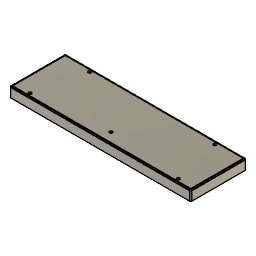
Like Vortex Core (Autodesk Fusion 360 design; units mm, degrees)
Autodesk Fusion 360 part; units mm, degrees
sketch "Sketch1" plane through (0, 0, 0) normal (0, 0, 1) x (1, 0, 0)
  line L0 (40.7197, 73.9331) -> (54.719, 73.9331)
  line L1 (19.0004, 40.8838) -> (5.0009, 40.8838)
  line L2 (173.782, 40.8838) -> (159.782, 40.8838)
  line L3 (238.075, 54.8831) -> (238.075, 40.8838)
  line L4 (54.719, 73.9331) -> (54.719, 59.9338)
  line L5 (245.219, 21.8336) -> (231.22, 21.8336)
  line L6 (40.7197, 59.9338) -> (40.7197, 73.9331)
  line L7 (211.882, 40.8838) -> (197.882, 40.8838)
  line L8 (59.7697, 73.9331) -> (73.769, 73.9331)
  line L9 (83.5822, 54.8831) -> (97.5815, 54.8831)
  line L10 (2.6197, 59.9338) -> (2.6197, 73.9331)
  line L11 (54.719, 59.9338) -> (40.7197, 59.9338)
  line L12 (173.782, 54.8831) -> (173.782, 40.8838)
  line L13 (64.5322, 40.8838) -> (64.5322, 54.8831)
  line L14 (83.5822, 40.8838) -> (83.5822, 54.8831)
  line L15 (21.6697, 59.9338) -> (21.6697, 73.9331)
  line L16 (159.782, 40.8838) -> (159.782, 54.8831)
  line L17 (26.4322, 40.8838) -> (26.4322, 54.8831)
  line L18 (97.5815, 40.8838) -> (83.5822, 40.8838)
  line L19 (245.219, 35.833) -> (245.219, 21.8336)
  line L20 (59.4815, 40.8838) -> (45.4822, 40.8838)
  line L21 (209.787, 35.833) -> (223.788, 35.833)
  line L22 (135.682, 40.8838) -> (121.682, 40.8838)
  line L23 (135.682, 54.8831) -> (135.682, 40.8838)
  line L24 (192.832, 54.8831) -> (192.832, 40.8838)
  line L25 (40.4315, 40.8838) -> (26.4322, 40.8838)
  line L26 (178.832, 40.8838) -> (178.832, 54.8831)
  line L27 (211.882, 54.8831) -> (211.882, 40.8838)
  line L28 (16.6192, 59.9338) -> (2.6196, 59.9338)
  line L29 (231.22, 35.833) -> (245.219, 35.833)
  line L30 (231.22, 21.8336) -> (231.22, 35.833)
  line L31 (16.6192, 73.9331) -> (16.6192, 59.9338)
  line L32 (238.075, 40.8838) -> (224.076, 40.8838)
  line L33 (154.732, 54.8831) -> (154.732, 40.8838)
  line L34 (154.732, 40.8838) -> (140.732, 40.8838)
  line L35 (223.788, 21.8336) -> (209.787, 21.8336)
  line L36 (64.5322, 54.8831) -> (78.5315, 54.8831)
  line L37 (197.882, 54.8831) -> (211.882, 54.8831)
  line L38 (5.0009, 54.8831) -> (19.0004, 54.8831)
  line L39 (21.6697, 73.9331) -> (35.669, 73.9331)
  line L40 (2.6197, 73.9331) -> (16.6192, 73.9331)
  line L41 (140.732, 40.8838) -> (140.732, 54.8831)
  line L42 (35.669, 73.9331) -> (35.669, 59.9338)
  line L43 (192.832, 40.8838) -> (178.832, 40.8838)
  line L44 (188.357, 21.8336) -> (188.357, 35.833)
  line L45 (197.882, 40.8838) -> (197.882, 54.8831)
  line L46 (102.632, 54.8831) -> (116.632, 54.8831)
  line L47 (178.832, 54.8831) -> (192.832, 54.8831)
  line L48 (59.4815, 54.8831) -> (59.4815, 40.8838)
  line L49 (224.076, 54.8831) -> (238.075, 54.8831)
  line L50 (19.0004, 54.8831) -> (19.0004, 40.8838)
  line L51 (133.587, 2.7836) -> (147.588, 2.7836)
  line L52 (45.4822, 40.8838) -> (45.4822, 54.8831)
  line L53 (116.632, 40.8838) -> (102.632, 40.8838)
  line L54 (5.0009, 40.8838) -> (5.0009, 54.8831)
  line L55 (159.782, 54.8831) -> (173.782, 54.8831)
  line L56 (26.4322, 54.8831) -> (40.4315, 54.8831)
  line L57 (97.5815, 54.8831) -> (97.5815, 40.8838)
  line L58 (223.788, 35.833) -> (223.788, 21.8336)
  line L59 (116.632, 54.8831) -> (116.632, 40.8838)
  line L60 (45.4822, 54.8831) -> (59.4815, 54.8831)
  line L61 (78.5315, 40.8838) -> (64.5322, 40.8838)
  line L62 (35.669, 59.9338) -> (21.6697, 59.9338)
  line L63 (209.787, 21.8336) -> (209.787, 35.833)
  line L64 (140.732, 54.8831) -> (154.732, 54.8831)
  line L65 (121.682, 40.8838) -> (121.682, 54.8831)
  line L66 (121.682, 54.8831) -> (135.682, 54.8831)
  line L67 (102.632, 40.8838) -> (102.632, 54.8831)
  line L68 (78.5315, 54.8831) -> (78.5315, 40.8838)
  line L69 (0.0951, 76.4575) -> (247.745, 76.4575)
  line L70 (40.4315, 54.8831) -> (40.4315, 40.8838)
  line L71 (224.076, 40.8838) -> (224.076, 54.8831)
  line L72 (0.0951, 0.2577) -> (0.0951, 76.4575)
  line L73 (247.745, 0.2577) -> (0.0951, 0.2577)
  line L74 (247.745, 76.4575) -> (247.745, 0.2577)
  line L75 (40.4315, 16.7831) -> (40.4315, 2.7836)
  line L76 (59.4815, 2.7836) -> (45.4822, 2.7836)
  line L77 (64.5322, 16.7831) -> (78.5315, 16.7831)
  line L78 (59.4815, 16.7831) -> (59.4815, 2.7836)
  line L79 (45.4822, 2.7836) -> (45.4822, 16.7831)
  line L80 (78.5315, 16.7831) -> (78.5315, 2.7836)
  line L81 (64.5322, 2.7836) -> (64.5322, 16.7831)
  line L82 (35.9572, 21.8336) -> (35.9572, 35.833)
  line L83 (202.357, 2.7836) -> (188.357, 2.7836)
  line L84 (19.0004, 2.7836) -> (5.0009, 2.7836)
  line L85 (90.726, 2.7836) -> (90.726, 16.7831)
  line L86 (5.0009, 16.7831) -> (19.0004, 16.7831)
  line L87 (26.4322, 2.7836) -> (26.4322, 16.7831)
  line L88 (88.0565, 35.833) -> (88.0565, 21.8336)
  line L89 (221.407, 16.7831) -> (221.407, 2.7836)
  line L90 (35.9572, 35.833) -> (49.9565, 35.833)
  line L91 (55.0072, 21.8336) -> (55.0072, 35.833)
  line L92 (147.588, 16.7831) -> (133.587, 16.7831)
  line L93 (45.4822, 16.7831) -> (59.4815, 16.7831)
  line L94 (78.5315, 2.7836) -> (64.5322, 2.7836)
  line L95 (40.4315, 2.7836) -> (26.4322, 2.7836)
  line L96 (19.0004, 16.7831) -> (19.0004, 2.7836)
  line L97 (5.0009, 2.7836) -> (5.0009, 16.7831)
  line L98 (26.4322, 16.7831) -> (40.4315, 16.7831)
  line L99 (9.762, 21.8336) -> (9.762, 35.833)
  line L100 (107.107, 35.833) -> (107.107, 21.8336)
  line L101 (88.0565, 21.8336) -> (74.0572, 21.8336)
  line L102 (49.9565, 21.8336) -> (35.9572, 21.8336)
  line L103 (90.726, 16.7831) -> (104.725, 16.7831)
  line L104 (183.307, 16.7831) -> (183.307, 2.7836)
  line L105 (107.107, 21.8336) -> (93.1072, 21.8336)
  line L106 (188.357, 16.7831) -> (202.357, 16.7831)
  line L107 (112.157, 35.833) -> (126.157, 35.833)
  line L108 (126.157, 21.8336) -> (112.157, 21.8336)
  line L109 (169.307, 2.7836) -> (169.307, 16.7831)
  line L110 (169.307, 16.7831) -> (183.307, 16.7831)
  line L111 (183.307, 2.7836) -> (169.307, 2.7836)
  line L112 (202.357, 16.7831) -> (202.357, 2.7836)
  line L113 (104.725, 2.7836) -> (90.726, 2.7836)
  line L114 (93.1072, 35.833) -> (107.107, 35.833)
  line L115 (131.207, 35.833) -> (145.207, 35.833)
  line L116 (150.257, 21.8336) -> (150.257, 35.833)
  line L117 (164.257, 35.833) -> (164.257, 21.8336)
  line L118 (188.357, 2.7836) -> (188.357, 16.7831)
  line L119 (207.407, 2.7836) -> (207.407, 16.7831)
  line L120 (169.307, 35.833) -> (183.307, 35.833)
  line L121 (69.0065, 21.8336) -> (55.0072, 21.8336)
  line L122 (49.9565, 35.833) -> (49.9565, 21.8336)
  line L123 (126.157, 35.833) -> (126.157, 21.8336)
  line L124 (164.257, 21.8336) -> (150.257, 21.8336)
  line L125 (145.207, 35.833) -> (145.207, 21.8336)
  line L126 (55.0072, 35.833) -> (69.0065, 35.833)
  line L127 (183.307, 35.833) -> (183.307, 21.8336)
  line L128 (112.157, 21.8336) -> (112.157, 35.833)
  line L129 (131.207, 21.8336) -> (131.207, 35.833)
  line L130 (104.725, 16.7831) -> (104.725, 2.7836)
  line L131 (93.1072, 21.8336) -> (93.1072, 35.833)
  line L132 (145.207, 21.8336) -> (131.207, 21.8336)
  line L133 (150.257, 35.833) -> (164.257, 35.833)
  line L134 (242.838, 2.7836) -> (228.837, 2.7836)
  line L135 (221.407, 2.7836) -> (207.407, 2.7836)
  line L136 (69.0065, 35.833) -> (69.0065, 21.8336)
  line L137 (74.0572, 35.833) -> (88.0565, 35.833)
  line L138 (207.407, 16.7831) -> (221.407, 16.7831)
  line L139 (207.119, 59.9338) -> (193.12, 59.9338)
  line L140 (202.357, 35.833) -> (202.357, 21.8336)
  line L141 (23.7629, 21.8336) -> (9.762, 21.8336)
  line L142 (116.918, 73.9331) -> (130.919, 73.9331)
  line L143 (183.307, 21.8336) -> (169.307, 21.8336)
  line L144 (228.837, 16.7831) -> (242.838, 16.7831)
  line L145 (228.837, 2.7836) -> (228.837, 16.7831)
  line L146 (188.357, 35.833) -> (202.357, 35.833)
  line L147 (23.7629, 35.833) -> (23.7629, 21.8336)
  line L148 (242.838, 16.7831) -> (242.838, 2.7836)
  line L149 (74.0572, 21.8336) -> (74.0572, 35.833)
  line L150 (9.762, 35.833) -> (23.7629, 35.833)
  line L151 (202.357, 21.8336) -> (188.357, 21.8336)
  line L152 (169.307, 21.8336) -> (169.307, 35.833)
  line L153 (188.069, 59.9338) -> (174.07, 59.9338)
  line L154 (169.019, 59.9338) -> (155.02, 59.9338)
  line L155 (97.8683, 59.9338) -> (97.8683, 73.9331)
  line L156 (135.97, 73.9331) -> (149.969, 73.9331)
  line L157 (169.019, 73.9331) -> (169.019, 59.9338)
  line L158 (226.169, 73.9331) -> (226.169, 59.9338)
  line L159 (73.769, 59.9338) -> (59.7697, 59.9338)
  line L160 (193.12, 73.9331) -> (207.119, 73.9331)
  line L161 (97.8683, 73.9331) -> (111.869, 73.9331)
  line L162 (155.02, 59.9338) -> (155.02, 73.9331)
  line L163 (111.869, 59.9338) -> (97.8683, 59.9338)
  line L164 (116.918, 59.9338) -> (116.918, 73.9331)
  line L165 (188.069, 73.9331) -> (188.069, 59.9338)
  line L166 (78.8197, 59.9338) -> (78.8197, 73.9331)
  line L167 (155.02, 73.9331) -> (169.019, 73.9331)
  line L168 (73.769, 73.9331) -> (73.769, 59.9338)
  line L169 (149.969, 73.9331) -> (149.969, 59.9338)
  line L170 (174.07, 73.9331) -> (188.069, 73.9331)
  line L171 (59.7697, 59.9338) -> (59.7697, 73.9331)
  line L172 (193.12, 59.9338) -> (193.12, 73.9331)
  line L173 (212.17, 59.9338) -> (212.17, 73.9331)
  line L174 (207.119, 73.9331) -> (207.119, 59.9338)
  line L175 (226.169, 59.9338) -> (212.17, 59.9338)
  line L176 (130.919, 59.9338) -> (116.918, 59.9338)
  line L177 (92.819, 59.9338) -> (78.8197, 59.9338)
  line L178 (130.919, 73.9331) -> (130.919, 59.9338)
  line L179 (149.969, 59.9338) -> (135.97, 59.9338)
  line L180 (78.8197, 73.9331) -> (92.819, 73.9331)
  line L181 (245.219, 59.9338) -> (231.22, 59.9338)
  line L182 (135.97, 59.9338) -> (135.97, 73.9331)
  line L183 (231.22, 73.9331) -> (245.219, 73.9331)
  line L184 (92.819, 73.9331) -> (92.819, 59.9338)
  line L185 (231.22, 59.9338) -> (231.22, 73.9331)
  line L186 (212.17, 73.9331) -> (226.169, 73.9331)
  line L187 (111.869, 73.9331) -> (111.869, 59.9338)
  line L188 (245.219, 73.9331) -> (245.219, 59.9338)
  line L189 (174.07, 59.9338) -> (174.07, 73.9331)
  line L190 (133.587, 16.7831) -> (133.587, 2.7836)
  line L191 (147.588, 2.7836) -> (147.588, 16.7831)
  line L192 (2.1383, 74.6931) -> (2.1383, 1.9601)
  line L193 (2.1383, 1.9601) -> (245.7226, 1.9601)
  line L194 (245.7226, 1.9601) -> (245.7226, 74.6931)
  line L195 (245.7226, 74.6931) -> (2.1383, 74.6931)
  line L196 (221.407, 9.3668) -> (228.837, 9.3668)
  line L197 (228.837, 9.3668) -> (228.837, 1.9601)
  line L198 (228.837, 1.9601) -> (221.407, 1.9601)
  line L199 (221.407, 1.9601) -> (221.407, 9.3668)
  line L200 (19.0004, 9.373) -> (26.4322, 9.373)
  line L201 (26.4322, 9.373) -> (26.4322, 1.9601)
  line L202 (26.4322, 1.9601) -> (19.0004, 1.9601)
  line L203 (19.0004, 1.9601) -> (19.0004, 9.373)
  circle A0 centre (123.9304, 14.9601) radius 3.5951
  line L204 (226.169, 68.4327) -> (231.22, 68.4327)
  line L205 (231.22, 68.4327) -> (231.22, 74.6931)
  line L206 (231.22, 74.6931) -> (226.169, 74.6931)
  line L207 (226.169, 74.6931) -> (226.169, 68.4327)
  line L208 (16.6192, 68.371) -> (21.6697, 68.371)
  line L209 (21.6697, 68.371) -> (21.6697, 74.6931)
  line L210 (21.6697, 74.6931) -> (16.6192, 74.6931)
  line L211 (16.6192, 74.6931) -> (16.6192, 68.371)
  line L212 (212.17, 68.3537) -> (207.119, 68.3537)
  line L213 (207.119, 73.9331) -> (207.119, 74.6931)
  line L214 (212.17, 73.9331) -> (212.17, 74.6931)
  line L215 (35.669, 68.3674) -> (40.7197, 68.3674)
  line L216 (40.7197, 73.9331) -> (40.7197, 74.6931)
  line L217 (35.669, 73.9331) -> (35.669, 74.6931)
  constraint perpendicular L51 L190
  constraint perpendicular L92 L191
  constraint perpendicular L73 L192
  constraint perpendicular L74 L193
  constraint perpendicular L193 L194
  constraint perpendicular L192 L195
  constraint parallel L69 L195
  constraint parallel L72 L192
  constraint parallel L73 L193
  constraint horizontal L196
  constraint vertical L197
  constraint horizontal L198
  constraint vertical L199
  constraint coincident L193 L197.end
  constraint coincident L89 L196.start
  constraint horizontal L200
  constraint vertical L201
  constraint horizontal L202
  constraint vertical L203
  constraint coincident L193 L201.end
  constraint coincident L96 L200.start
  constraint horizontal L204
  constraint vertical L205
  constraint horizontal L206
  constraint vertical L207
  constraint coincident L195 L205.end
  constraint coincident L158 L204.start
  constraint horizontal L208
  constraint vertical L209
  constraint horizontal L210
  constraint vertical L211
  constraint coincident L195 L209.end
  constraint coincident L31 L208.start
  constraint coincident L173 L212.start
  constraint coincident L174 L212.end
  constraint perpendicular L174 L212
  constraint coincident L195 L213.end
  constraint perpendicular L195 L213
  constraint coincident L195 L214.end
  constraint perpendicular L195 L214
  constraint coincident L42 L215.start
  constraint coincident L6 L215.end
  constraint perpendicular L6 L215
  constraint coincident L195 L216.end
  constraint perpendicular L195 L216
  constraint coincident L195 L217.end
  constraint perpendicular L195 L217
extrude "Extrude1" add sketch "Sketch1" against normal blind 1.5 contours L0 L4 L6 L10 L11 L15 L28 L31 L40 L42 L62 L75 L84 L86 L87 L89 L95 L96 L97 L98 L119 L134 L135 L138 L139 L144 L145 L148 L158 L160 L172 L173 L174 L175 L181 L183 L185 L188 L192 L193 L194 L195 L196 L197 L199 L200 L201 L203 L204 L205 L208 L211 L212 L213 L215 L216 | L6 L42 L195 L215 L216 L217 | L173 L174 L195 L212 L213 L214 | L39 L195 L209 L217 | L186 L195 L207 L214 | L15 L31 L195 L208 L209 L210 L211 | L158 L185 L195 L204 L205 L206 L207 | L87 L96 L193 L200 L201 L202 L203 | L89 L145 L193 L196 L197 L198 L199 | L69 L72 L73 L74 | A0 makes body 1
extrude "Extrude2" add sketch "Sketch1" along normal blind 3.5 contours L69 L72 L73 L74 bodies 1
extrude "Extrude6" add 1 faces at (0.7761, 50.4694, 3.5) along direction (0, 0, 1) blind 7.5 draft 10 on bodies 1 bodies 1
sketch "Sketch6" plane through (0, 0, -1.5) normal (0, 0, -1) x (1, 0, 0)
  line L0 (147.588, -2.7836) -> (147.588, -16.7831)
  line L1 (147.588, -16.7831) -> (133.587, -16.7831)
  line L2 (133.587, -16.7831) -> (133.587, -2.7836)
  line L3 (133.587, -2.7836) -> (147.588, -2.7836)
  line L4 (174.07, -59.9338) -> (188.069, -59.9338)
  line L5 (188.069, -59.9338) -> (188.069, -73.9331)
  line L6 (188.069, -73.9331) -> (174.07, -73.9331)
  line L7 (174.07, -73.9331) -> (174.07, -59.9338)
  line L8 (245.219, -73.9331) -> (231.22, -73.9331)
  line L9 (231.22, -73.9331) -> (231.22, -59.9338)
  line L10 (231.22, -59.9338) -> (245.219, -59.9338)
  line L11 (245.219, -59.9338) -> (245.219, -73.9331)
  line L12 (111.869, -73.9331) -> (97.8683, -73.9331)
  line L13 (97.8683, -73.9331) -> (97.8683, -59.9338)
  line L14 (97.8683, -59.9338) -> (111.869, -59.9338)
  line L15 (111.869, -59.9338) -> (111.869, -73.9331)
  line L16 (212.17, -73.9331) -> (212.17, -59.9338)
  line L17 (212.17, -59.9338) -> (226.169, -59.9338)
  line L18 (226.169, -59.9338) -> (226.169, -73.9331)
  line L19 (226.169, -73.9331) -> (212.17, -73.9331)
  line L20 (92.819, -73.9331) -> (78.8197, -73.9331)
  line L21 (78.8197, -73.9331) -> (78.8197, -59.9338)
  line L22 (78.8197, -59.9338) -> (92.819, -59.9338)
  line L23 (92.819, -59.9338) -> (92.819, -73.9331)
  line L24 (135.97, -59.9338) -> (149.969, -59.9338)
  line L25 (149.969, -59.9338) -> (149.969, -73.9331)
  line L26 (149.969, -73.9331) -> (135.97, -73.9331)
  line L27 (135.97, -73.9331) -> (135.97, -59.9338)
  line L28 (130.919, -73.9331) -> (116.918, -73.9331)
  line L29 (116.918, -73.9331) -> (116.918, -59.9338)
  line L30 (116.918, -59.9338) -> (130.919, -59.9338)
  line L31 (130.919, -59.9338) -> (130.919, -73.9331)
  line L32 (207.119, -73.9331) -> (193.12, -73.9331)
  line L33 (193.12, -73.9331) -> (193.12, -59.9338)
  line L34 (193.12, -59.9338) -> (207.119, -59.9338)
  line L35 (207.119, -59.9338) -> (207.119, -73.9331)
  line L36 (59.7697, -59.9338) -> (73.769, -59.9338)
  line L37 (73.769, -59.9338) -> (73.769, -73.9331)
  line L38 (73.769, -73.9331) -> (59.7697, -73.9331)
  line L39 (59.7697, -73.9331) -> (59.7697, -59.9338)
  line L40 (155.02, -73.9331) -> (155.02, -59.9338)
  line L41 (155.02, -59.9338) -> (169.019, -59.9338)
  line L42 (169.019, -59.9338) -> (169.019, -73.9331)
  line L43 (169.019, -73.9331) -> (155.02, -73.9331)
  line L44 (169.307, -21.8336) -> (183.307, -21.8336)
  line L45 (183.307, -21.8336) -> (183.307, -35.833)
  line L46 (183.307, -35.833) -> (169.307, -35.833)
  line L47 (169.307, -35.833) -> (169.307, -21.8336)
  line L48 (202.357, -21.8336) -> (202.357, -35.833)
  line L49 (202.357, -35.833) -> (188.357, -35.833)
  line L50 (188.357, -35.833) -> (188.357, -21.8336)
  line L51 (188.357, -21.8336) -> (202.357, -21.8336)
  line L52 (9.762, -35.833) -> (9.762, -21.8336)
  line L53 (9.762, -21.8336) -> (23.7629, -21.8336)
  line L54 (23.7629, -21.8336) -> (23.7629, -35.833)
  line L55 (23.7629, -35.833) -> (9.762, -35.833)
  line L56 (74.0572, -21.8336) -> (88.0565, -21.8336)
  line L57 (88.0565, -21.8336) -> (88.0565, -35.833)
  line L58 (88.0565, -35.833) -> (74.0572, -35.833)
  line L59 (74.0572, -35.833) -> (74.0572, -21.8336)
  line L60 (242.838, -16.7831) -> (228.837, -16.7831)
  line L61 (228.837, -16.7831) -> (228.837, -2.7836)
  line L62 (228.837, -2.7836) -> (242.838, -2.7836)
  line L63 (242.838, -2.7836) -> (242.838, -16.7831)
  line L64 (207.407, -16.7831) -> (207.407, -2.7836)
  line L65 (207.407, -2.7836) -> (221.407, -2.7836)
  line L66 (221.407, -2.7836) -> (221.407, -16.7831)
  line L67 (221.407, -16.7831) -> (207.407, -16.7831)
  line L68 (69.0065, -35.833) -> (55.0072, -35.833)
  line L69 (55.0072, -35.833) -> (55.0072, -21.8336)
  line L70 (55.0072, -21.8336) -> (69.0065, -21.8336)
  line L71 (69.0065, -21.8336) -> (69.0065, -35.833)
  line L72 (121.682, -54.8831) -> (121.682, -40.8838)
  line L73 (121.682, -40.8838) -> (135.682, -40.8838)
  line L74 (135.682, -40.8838) -> (135.682, -54.8831)
  line L75 (135.682, -54.8831) -> (121.682, -54.8831)
  line L76 (45.4822, -16.7831) -> (45.4822, -2.7836)
  line L77 (45.4822, -2.7836) -> (59.4815, -2.7836)
  line L78 (59.4815, -2.7836) -> (59.4815, -16.7831)
  line L79 (59.4815, -16.7831) -> (45.4822, -16.7831)
  line L80 (183.307, -2.7836) -> (183.307, -16.7831)
  line L81 (183.307, -16.7831) -> (169.307, -16.7831)
  line L82 (169.307, -16.7831) -> (169.307, -2.7836)
  line L83 (169.307, -2.7836) -> (183.307, -2.7836)
  line L84 (93.1072, -21.8336) -> (107.107, -21.8336)
  line L85 (107.107, -21.8336) -> (107.107, -35.833)
  line L86 (107.107, -35.833) -> (93.1072, -35.833)
  line L87 (93.1072, -35.833) -> (93.1072, -21.8336)
  line L88 (45.4822, -54.8831) -> (45.4822, -40.8838)
  line L89 (45.4822, -40.8838) -> (59.4815, -40.8838)
  line L90 (59.4815, -40.8838) -> (59.4815, -54.8831)
  line L91 (59.4815, -54.8831) -> (45.4822, -54.8831)
  line L92 (40.4315, -54.8831) -> (26.4322, -54.8831)
  line L93 (26.4322, -54.8831) -> (26.4322, -40.8838)
  line L94 (26.4322, -40.8838) -> (40.4315, -40.8838)
  line L95 (40.4315, -40.8838) -> (40.4315, -54.8831)
  line L96 (231.22, -21.8336) -> (245.219, -21.8336)
  line L97 (245.219, -21.8336) -> (245.219, -35.833)
  line L98 (245.219, -35.833) -> (231.22, -35.833)
  line L99 (231.22, -35.833) -> (231.22, -21.8336)
  line L100 (104.725, -16.7831) -> (90.726, -16.7831)
  line L101 (90.726, -16.7831) -> (90.726, -2.7836)
  line L102 (90.726, -2.7836) -> (104.725, -2.7836)
  line L103 (104.725, -2.7836) -> (104.725, -16.7831)
  line L104 (150.257, -35.833) -> (150.257, -21.8336)
  line L105 (150.257, -21.8336) -> (164.257, -21.8336)
  line L106 (164.257, -21.8336) -> (164.257, -35.833)
  line L107 (164.257, -35.833) -> (150.257, -35.833)
  line L108 (54.719, -59.9338) -> (54.719, -73.9331)
  line L109 (54.719, -73.9331) -> (40.7197, -73.9331)
  line L110 (40.7197, -73.9331) -> (40.7197, -59.9338)
  line L111 (40.7197, -59.9338) -> (54.719, -59.9338)
  line L112 (35.669, -59.9338) -> (35.669, -73.9331)
  line L113 (35.669, -73.9331) -> (21.6697, -73.9331)
  line L114 (21.6697, -73.9331) -> (21.6697, -59.9338)
  line L115 (21.6697, -59.9338) -> (35.669, -59.9338)
  line L116 (2.6197, -73.9331) -> (2.6197, -59.9338)
  line L117 (2.6197, -59.9338) -> (16.6192, -59.9338)
  line L118 (16.6192, -59.9338) -> (16.6192, -73.9331)
  line L119 (16.6192, -73.9331) -> (2.6197, -73.9331)
  line L120 (159.782, -54.8831) -> (159.782, -40.8838)
  line L121 (159.782, -40.8838) -> (173.782, -40.8838)
  line L122 (173.782, -40.8838) -> (173.782, -54.8831)
  line L123 (173.782, -54.8831) -> (159.782, -54.8831)
  line L124 (145.207, -21.8336) -> (145.207, -35.833)
  line L125 (145.207, -35.833) -> (131.207, -35.833)
  line L126 (131.207, -35.833) -> (131.207, -21.8336)
  line L127 (131.207, -21.8336) -> (145.207, -21.8336)
  line L128 (49.9565, -35.833) -> (35.9572, -35.833)
  line L129 (35.9572, -35.833) -> (35.9572, -21.8336)
  line L130 (35.9572, -21.8336) -> (49.9565, -21.8336)
  line L131 (49.9565, -21.8336) -> (49.9565, -35.833)
  line L132 (178.832, -54.8831) -> (178.832, -40.8838)
  line L133 (178.832, -40.8838) -> (192.832, -40.8838)
  line L134 (192.832, -40.8838) -> (192.832, -54.8831)
  line L135 (192.832, -54.8831) -> (178.832, -54.8831)
  line L136 (5.0009, -40.8838) -> (19.0004, -40.8838)
  line L137 (19.0004, -40.8838) -> (19.0004, -54.8831)
  line L138 (19.0004, -54.8831) -> (5.0009, -54.8831)
  line L139 (5.0009, -54.8831) -> (5.0009, -40.8838)
  line L140 (224.076, -40.8838) -> (238.075, -40.8838)
  line L141 (238.075, -40.8838) -> (238.075, -54.8831)
  line L142 (238.075, -54.8831) -> (224.076, -54.8831)
  line L143 (224.076, -54.8831) -> (224.076, -40.8838)
  line L144 (112.157, -21.8336) -> (126.157, -21.8336)
  line L145 (126.157, -21.8336) -> (126.157, -35.833)
  line L146 (126.157, -35.833) -> (112.157, -35.833)
  line L147 (112.157, -35.833) -> (112.157, -21.8336)
  line L148 (5.0009, -2.7836) -> (19.0004, -2.7836)
  line L149 (19.0004, -2.7836) -> (19.0004, -16.7831)
  line L150 (19.0004, -16.7831) -> (5.0009, -16.7831)
  line L151 (5.0009, -16.7831) -> (5.0009, -2.7836)
  line L152 (78.5315, -2.7836) -> (78.5315, -16.7831)
  line L153 (78.5315, -16.7831) -> (64.5322, -16.7831)
  line L154 (64.5322, -16.7831) -> (64.5322, -2.7836)
  line L155 (64.5322, -2.7836) -> (78.5315, -2.7836)
  line L156 (102.632, -40.8838) -> (116.632, -40.8838)
  line L157 (116.632, -40.8838) -> (116.632, -54.8831)
  line L158 (116.632, -54.8831) -> (102.632, -54.8831)
  line L159 (102.632, -54.8831) -> (102.632, -40.8838)
  line L160 (197.882, -40.8838) -> (211.882, -40.8838)
  line L161 (211.882, -40.8838) -> (211.882, -54.8831)
  line L162 (211.882, -54.8831) -> (197.882, -54.8831)
  line L163 (197.882, -54.8831) -> (197.882, -40.8838)
  line L164 (97.5815, -54.8831) -> (83.5822, -54.8831)
  line L165 (83.5822, -54.8831) -> (83.5822, -40.8838)
  line L166 (83.5822, -40.8838) -> (97.5815, -40.8838)
  line L167 (97.5815, -40.8838) -> (97.5815, -54.8831)
  line L168 (26.4322, -16.7831) -> (26.4322, -2.7836)
  line L169 (26.4322, -2.7836) -> (40.4315, -2.7836)
  line L170 (40.4315, -2.7836) -> (40.4315, -16.7831)
  line L171 (40.4315, -16.7831) -> (26.4322, -16.7831)
  line L172 (188.357, -2.7836) -> (202.357, -2.7836)
  line L173 (202.357, -2.7836) -> (202.357, -16.7831)
  line L174 (202.357, -16.7831) -> (188.357, -16.7831)
  line L175 (188.357, -16.7831) -> (188.357, -2.7836)
  line L176 (209.787, -21.8336) -> (223.788, -21.8336)
  line L177 (223.788, -21.8336) -> (223.788, -35.833)
  line L178 (223.788, -35.833) -> (209.787, -35.833)
  line L179 (209.787, -35.833) -> (209.787, -21.8336)
  line L180 (78.5315, -54.8831) -> (64.5322, -54.8831)
  line L181 (64.5322, -54.8831) -> (64.5322, -40.8838)
  line L182 (64.5322, -40.8838) -> (78.5315, -40.8838)
  line L183 (78.5315, -40.8838) -> (78.5315, -54.8831)
  line L184 (140.732, -54.8831) -> (140.732, -40.8838)
  line L185 (140.732, -40.8838) -> (154.732, -40.8838)
  line L186 (154.732, -40.8838) -> (154.732, -54.8831)
  line L187 (154.732, -54.8831) -> (140.732, -54.8831)
  line L188 (0.0951, -76.4575) -> (247.745, -76.4575)
  line L189 (247.745, -76.4575) -> (247.745, -0.2577)
  line L190 (247.745, -0.2577) -> (0.0951, -0.2577)
  line L191 (0.0951, -0.2577) -> (0.0951, -76.4575)
  line L192 (0.0951, -76.4575) -> (247.745, -76.4575)
  line L193 (247.745, -76.4575) -> (247.745, -0.2577)
  line L194 (247.745, -0.2577) -> (0.0951, -0.2577)
  line L195 (0.0951, -0.2577) -> (0.0951, -76.4575)
  constraint horizontal L192
  constraint vertical L193
  constraint horizontal L194
  constraint vertical L195
  constraint coincident L189.end L190.start
  constraint coincident L188.start L191.end
extrude "Extrude7" cut sketch "Sketch6" against normal blind 40 contours L0 L1 L2 L3 | L4 L5 L6 L7 | L8 L9 L10 L11 | L12 L13 L14 L15 | L16 L17 L18 L19 | L20 L21 L22 L23 | L24 L25 L26 L27 | L28 L29 L30 L31 | L32 L33 L34 L35 | L36 L37 L38 L39 | L40 L41 L42 L43 | L44 L45 L46 L47 | L48 L49 L50 L51 | L52 L53 L54 L55 | L56 L57 L58 L59 | L60 L61 L62 L63 | L64 L65 L66 L67 | L68 L69 L70 L71 | L72 L73 L74 L75 | L76 L77 L78 L79 | L80 L81 L82 L83 | L84 L85 L86 L87 | L88 L89 L90 L91 | L92 L93 L94 L95 | L96 L97 L98 L99 | L100 L101 L102 L103 | L104 L105 L106 L107 | L108 L109 L110 L111 | L112 L113 L114 L115 | L116 L117 L118 L119 | L120 L121 L122 L123 | L124 L125 L126 L127 | L128 L129 L130 L131 | L132 L133 L134 L135 | L136 L137 L138 L139 | L140 L141 L142 L143 | L144 L145 L146 L147 | L148 L149 L150 L151 | L152 L153 L154 L155 | L156 L157 L158 L159 | L160 L161 L162 L163 | L164 L165 L166 L167 | L168 L169 L170 L171 | L172 L173 L174 L175 | L176 L177 L178 L179 | L180 L181 L182 L183 | L184 L185 L186 L187 | L188 L189 L190 L191 L192 L193 L194 L195 keep common part bodies 1
extrude "Extrude4" add sketch "Sketch1" along normal blind 11 contours L6 L42 L195 L215 L216 L217 | L173 L174 L195 L212 L213 L214 | L87 L96 L193 L200 L201 L202 L203 | L89 L145 L193 L196 L197 L198 L199 | A0 bodies 1
sketch "Sketch5" plane through (0, 0, 11) normal (0, 0, 1) x (-1, 0, 0)
  line L0 (-228.837, -3.2826) -> (-228.837, -9.3668)
  line L1 (-228.837, -9.3668) -> (-221.407, -9.3668)
  line L2 (-221.407, -9.3668) -> (-221.407, -3.2826)
  line L3 (-26.4322, -3.2826) -> (-26.4322, -9.373)
  line L4 (-26.4322, -9.373) -> (-19.0004, -9.373)
  line L5 (-19.0004, -9.373) -> (-19.0004, -3.2826)
  line L6 (-247.745, -76.4575) -> (-0.0951, -76.4575)
  line L7 (-0.0951, -76.4575) -> (-0.0951, -0.2577)
  line L8 (-0.0951, -0.2577) -> (-247.745, -0.2577)
  line L9 (-247.745, -0.2577) -> (-247.745, -76.4575)
  line L10 (-2.1277, -74.4552) -> (-245.6919, -74.4552)
  line L11 (-245.6919, -74.4552) -> (-245.6919, -2.3183)
  line L12 (-245.6919, -2.3183) -> (-2.1277, -2.3183)
  line L13 (-2.1277, -2.3183) -> (-2.1277, -74.4552)
  line L14 (-19.0004, -3.2826) -> (-3.4607, -3.2826)
  line L15 (-3.4607, -3.2826) -> (-3.4607, -73.3706)
  line L16 (-40.7197, -73.3706) -> (-207.119, -73.3706)
  line L17 (-244.4001, -73.3706) -> (-244.4001, -3.2826)
  line L18 (-244.4001, -3.2826) -> (-228.837, -3.2826)
  line L19 (-221.407, -3.2826) -> (-26.4322, -3.2826)
  line L20 (-207.119, -73.3706) -> (-207.119, -68.3537)
  line L21 (-207.119, -68.3537) -> (-212.17, -68.3537)
  line L22 (-212.17, -68.3537) -> (-212.17, -73.3706)
  line L23 (-212.17, -73.3706) -> (-244.4001, -73.3706)
  line L24 (-3.4607, -73.3706) -> (-35.669, -73.3706)
  line L25 (-35.669, -73.3706) -> (-35.669, -68.3674)
  line L26 (-35.669, -68.3674) -> (-40.7197, -68.3674)
  line L27 (-40.7197, -68.3674) -> (-40.7197, -73.3706)
  constraint horizontal L10
  constraint vertical L11
  constraint horizontal L12
  constraint vertical L13
extrude "Extrude5" add sketch "Sketch5" along normal blind 1.5 contours L6 L7 L8 L9 bodies 1
fillet "Fillet3" radius 1.5 4 edges at (0.0951, 76.4575, 5.5) (0.0951, 0.2577, 5.5) (247.745, 0.2577, 5.5) (247.745, 76.4575, 5.5) on bodies 1
fillet "Fillet4" radius 19.75 12 edges at (123.9196, 1.9601, 3.5) (237.2798, 1.9601, 3.5) (245.7226, 38.3266, 3.5) (228.9463, 74.6931, 3.5) (123.9194, 74.6931, 3.5) (18.9036, 74.6931, 3.5) (228.9463, 74.6931, 3.5) (123.9194, 74.6931, 3.5) (18.9036, 74.6931, 3.5) (2.1383, 38.3266, 3.5) (18.9036, 74.6931, 3.5) (10.5693, 1.9601, 3.5) on bodies 1
sketch "Sketch7" plane through (0, 76.4575, 0) normal (0, 1, 0) x (-1, 0, 0)
  line L0 (-246.245, 12.5) -> (-246.245, -1.5)
  line L1 (-246.245, -1.5) -> (-1.5951, -1.5)
  line L2 (-1.5951, -1.5) -> (-1.5951, 12.5)
  line L3 (-1.5951, 12.5) -> (-246.245, 12.5)
  line L4 (-23.4098, 9) -> (-14.4098, 9)
  line L5 (-14.4098, 9) -> (-14.4098, 5.5)
  line L6 (-14.4098, 5.5) -> (-23.4098, 5.5)
  line L7 (-23.4098, 5.5) -> (-23.4098, 9)
  line L8 (-245.6919, 11) -> (-2.1277, 11)
  dimension "d27" = 3.5
  constraint horizontal L4
  constraint vertical L5
  constraint horizontal L6
  constraint vertical L7
  measures "d27" distance of L4.start L6.end
extrude "Extrude8" cut sketch "Sketch7" against normal blind 12 contours L4 L5 L6 L7 bodies 1
fillet "Fillet5" radius 1.75 4 edges at (14.4098, 75.0904, 9) (14.4098, 75.3989, 5.5) (23.4098, 75.3989, 5.5) (23.4098, 75.0904, 9) on bodies 1
sketch "Sketch8" plane through (0, 0, 12.5) normal (0, 0, 1) x (-1, 0, 0)
  line L0 (-245.6919, -2.3183) -> (-2.1277, -2.3183)
  line L1 (-2.1277, -2.3183) -> (-2.1277, -74.4552)
  line L2 (-2.1277, -74.4552) -> (-245.6919, -74.4552)
  line L3 (-245.6919, -74.4552) -> (-245.6919, -2.3183)
  arc A0 (-247.745, -74.9575) -> (-246.245, -76.4575) centre (-246.245, -74.9575) ccw
  line L4 (-246.245, -76.4575) -> (-1.5951, -76.4575)
  arc A1 (-1.5951, -76.4575) -> (-0.0951, -74.9575) centre (-1.5951, -74.9575) ccw
  line L5 (-0.0951, -74.9575) -> (-0.0951, -1.7577)
  arc A2 (-0.0951, -1.7577) -> (-1.5951, -0.2577) centre (-1.5951, -1.7577) ccw
  line L6 (-1.5951, -0.2577) -> (-246.245, -0.2577)
  arc A3 (-246.245, -0.2577) -> (-247.745, -1.7577) centre (-246.245, -1.7577) ccw
  line L7 (-247.745, -1.7577) -> (-247.745, -74.9575)
  line L8 (-30.4503, -74.4552) -> (-7.3693, -74.4552)
  line L9 (-7.3693, -74.4552) -> (-7.3693, -67.7003)
  line L10 (-7.3693, -67.7003) -> (-30.4503, -67.7003)
  line L11 (-30.4503, -67.7003) -> (-30.4503, -74.4552)
extrude "Extrude9" cut sketch "Sketch8" against normal blind 12 contours L2 L8 L9 L10 L11 bodies 1
fillet "Fillet6" radius 0.75 4 edges at (2.1277, 74.4552, 11.75) (245.6919, 74.4552, 11.75) (245.6919, 2.3183, 11.75) (2.1277, 2.3183, 11.75) on bodies 1
fillet "Fillet7" radius 1 12 edges at (2.1383, 74.6931, 0.886) (2.2134, 74.6179, 3.4934) (2.9495, 73.8818, 8.1008) (2.1383, 1.9601, 0.886) (2.2134, 2.0353, 3.4934) (2.9495, 2.7714, 8.1008) (245.7226, 1.9601, 0.886) (245.6474, 2.0353, 3.4934) (244.9114, 2.7714, 8.1008) (245.7226, 74.6931, 0.886) (245.6474, 74.6179, 3.4934) (244.9114, 73.8818, 8.1008) on bodies 1
sketch "Sketch11" plane through (0, 0, 12.5) normal (0, 0, 1) x (-1, 0, 0)
  line L0 (-244.9419, -2.3183) -> (-2.8777, -2.3183)
  arc A0 (-2.1277, -3.0683) -> (-2.8777, -2.3183) centre (-2.8777, -3.0683) ccw
  line L1 (-2.1277, -3.0683) -> (-2.1277, -73.7052)
  arc A1 (-2.8777, -74.4552) -> (-2.1277, -73.7052) centre (-2.8777, -73.7052) ccw
  line L2 (-2.8777, -74.4552) -> (-244.9419, -74.4552)
  arc A2 (-245.6919, -73.7052) -> (-244.9419, -74.4552) centre (-244.9419, -73.7052) ccw
  line L3 (-245.6919, -73.7052) -> (-245.6919, -3.0683)
  arc A3 (-244.9419, -2.3183) -> (-245.6919, -3.0683) centre (-244.9419, -3.0683) ccw
  arc A4 (-247.745, -74.9575) -> (-246.245, -76.4575) centre (-246.245, -74.9575) ccw
  line L4 (-246.245, -76.4575) -> (-1.5951, -76.4575)
  arc A5 (-1.5951, -76.4575) -> (-0.0951, -74.9575) centre (-1.5951, -74.9575) ccw
  line L5 (-0.0951, -74.9575) -> (-0.0951, -1.7577)
  arc A6 (-0.0951, -1.7577) -> (-1.5951, -0.2577) centre (-1.5951, -1.7577) ccw
  line L6 (-1.5951, -0.2577) -> (-246.245, -0.2577)
  arc A7 (-246.245, -0.2577) -> (-247.745, -1.7577) centre (-246.245, -1.7577) ccw
  line L7 (-247.745, -1.7577) -> (-247.745, -74.9575)
extrude "Extrude10" add sketch "Sketch11" against normal blind 1.5 separate body contours L0 A0 L1 A1 L2 A2 L3 A3 makes body 2
sketch "Sketch12" plane through (0, 0, 11) normal (0, 0, -1) x (1, 0, 0)
  arc A0 (2.8777, -2.3183) -> (2.1277, -3.0683) centre (2.8777, -3.0683) ccw
  line L0 (2.1277, -3.0683) -> (2.1277, -73.7052)
  arc A1 (2.1277, -73.7052) -> (2.8777, -74.4552) centre (2.8777, -73.7052) ccw
  line L1 (2.8777, -74.4552) -> (244.9419, -74.4552)
  arc A2 (244.9419, -74.4552) -> (245.6919, -73.7052) centre (244.9419, -73.7052) ccw
  line L2 (245.6919, -73.7052) -> (245.6919, -3.0683)
  arc A3 (245.6919, -3.0683) -> (244.9419, -2.3183) centre (244.9419, -3.0683) ccw
  line L3 (244.9419, -2.3183) -> (2.8777, -2.3183)
  line L4 (30.4098, -74.4552) -> (7.4098, -74.4552)
  line L5 (7.4098, -74.4552) -> (7.4098, -37.4552)
  line L6 (7.4098, -37.4552) -> (30.4098, -37.4552)
  line L7 (30.4098, -37.4552) -> (30.4098, -74.4552)
  line L8 (32.3439, -74.4552) -> (5.4296, -74.4552)
  line L9 (5.4296, -74.4552) -> (5.4296, -35.2609)
  line L10 (5.4296, -35.2609) -> (32.3439, -35.2609)
  line L11 (32.3439, -35.2609) -> (32.3439, -74.4552)
  line L12 (7.4098, -37.4552) -> (7.4098, -35.2609)
  line L13 (30.4098, -37.4552) -> (30.4098, -35.2609)
  dimension "d44" = 23
  dimension "d45" = 37
  constraint horizontal L4
  constraint vertical L5
  constraint horizontal L6
  constraint vertical L7
  constraint coincident L1 L4.start
  constraint horizontal L8
  constraint vertical L9
  constraint horizontal L10
  constraint vertical L11
  constraint coincident L1 L8.start
  constraint coincident L10 L12.end
  constraint perpendicular L10 L12
  constraint coincident L10 L13.end
  constraint perpendicular L10 L13
  measures "d44" distance of L4.start L4.end
  measures "d45" distance of L4.start L6.end
extrude "Extrude11" add sketch "Sketch12" along normal blind 2 contours L6 L10 L12 L13 bodies 2
fillet "Fillet10" radius 1 8 edges at (247.3057, 76.0182, 12.5) (123.92, 76.4575, 12.5) (0.5344, 76.0182, 12.5) (0.0951, 38.3576, 12.5) (0.5344, 0.697, 12.5) (123.92, 0.2577, 12.5) (247.3057, 0.697, 12.5) (247.745, 38.3576, 12.5) on bodies 1
fillet "Fillet11" radius 1 5 edges at (120.5786, 16.2602, 0) (225.122, 9.3668, 0) (22.7163, 9.373, 0) (209.6445, 68.3537, 0) (38.1944, 68.3674, 0) on bodies 1
fillet "Fillet12" radius 0.75 24 edges at (212.17, 73.8818, 8.1008) (212.17, 74.6179, 3.4934) (212.17, 74.6931, 0.886) (207.119, 74.6931, 0.886) (207.119, 74.6179, 3.4934) (207.119, 73.8818, 8.1008) (40.7197, 73.8818, 8.1008) (40.7197, 74.6179, 3.4934) (40.7197, 74.6931, 0.886) (35.669, 74.6931, 0.886) (35.669, 74.6179, 3.4934) (35.669, 73.8818, 8.1008) (26.4322, 1.9601, 0.886) (26.4322, 2.0353, 3.4934) (26.4322, 2.7714, 8.1008) (19.0004, 2.7714, 8.1008) (19.0004, 2.0353, 3.4934) (19.0004, 1.9601, 0.886) (221.407, 2.7714, 8.1008) (221.407, 2.0353, 3.4934) (221.407, 1.9601, 0.886) (228.837, 1.9601, 0.886) (228.837, 2.0353, 3.4934) (228.837, 2.7714, 8.1008) on bodies 1
fillet "Fillet13" radius 1.5 5 edges at (18.9098, 35.2609, 11) (7.4098, 36.3581, 11) (30.4098, 36.3581, 11) (30.4098, 35.2609, 10) (7.4098, 35.2609, 10) on bodies 2
fillet "Fillet14" radius 0.5 8 edges at (247.3057, 76.0182, -1.5) (247.745, 38.3576, -1.5) (247.3057, 0.697, -1.5) (123.92, 0.2577, -1.5) (0.5344, 0.697, -1.5) (0.0951, 38.3576, -1.5) (0.5344, 76.0182, -1.5) (123.92, 76.4575, -1.5) on bodies 1
hole "Hole2" at (225.2794, 5.7275, 12.5) direction (0, 0, -1) diameter 2 depth 9 tip angle 180 countersink diameter 4 countersink angle 90 bodies 1 2
hole "Hole3" at (38.229, 71.3939, 12.5) direction (0, 0, -1) diameter 2 depth 9 tip angle 180 countersink diameter 4 countersink angle 90 bodies 1 2
hole "Hole4" at (22.7627, 5.7613, 12.5) direction (0, 0, -1) diameter 2 depth 9 tip angle 180 countersink diameter 4 countersink angle 90 bodies 1 2
hole "Hole5" at (209.6639, 71.2524, 12.5) direction (0, 0, -1) diameter 2 depth 9 tip angle 180 countersink diameter 4 countersink angle 90 bodies 1 2
hole "Hole6" at (123.9894, 14.937, 12.5) direction (0, 0, -1) diameter 2 depth 9 tip angle 180 countersink diameter 4 countersink angle 90 bodies 1 2
named bodies: "Shell", "Bottom Plate"
